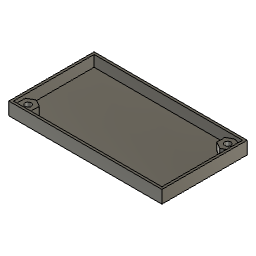
Assemblage v5 (Autodesk Fusion 360 archive; units mm, degrees)
design "Bas"
part number: Configuration1
Autodesk Fusion 360 part; units mm, degrees
sketch "Sketch1" plane through (0, 0, 0) normal (0, 0, 1) x (1, 0, 0)
  line L0 (0, 0) -> (79, 0)
  line L1 (79, 0) -> (79, 44)
  line L2 (79, 44) -> (0, 44)
  line L3 (0, 44) -> (0, 0)
  line L4 (1.2, 1.2) -> (77.8, 1.2)
  line L5 (77.8, 1.2) -> (77.8, 42.8)
  line L6 (77.8, 42.8) -> (1.2, 42.8)
  line L7 (1.2, 42.8) -> (1.2, 1.2)
  line L8 (2, 42) -> (77, 42) construction
  line L9 (77, 42) -> (77, 2) construction
  line L10 (77, 2) -> (2, 2) construction
  line L11 (2, 2) -> (2, 42) construction
  circle A0 centre (74, 39) radius 1.6
  circle A1 centre (5, 5) radius 1.6
  line L12 (74, 42.2332) -> (71.2, 40.6166)
  line L13 (71.2, 40.6166) -> (71.2, 37.3834)
  line L14 (71.2, 37.3834) -> (74, 35.7668)
  line L15 (74, 35.7668) -> (76.8, 37.3834)
  line L16 (76.8, 37.3834) -> (76.8, 40.6166)
  line L17 (76.8, 40.6166) -> (74, 42.2332)
  line L18 (5, 8.2332) -> (2.2, 6.6166)
  line L19 (2.2, 6.6166) -> (2.2, 3.3834)
  line L20 (2.2, 3.3834) -> (5, 1.7668)
  line L21 (5, 1.7668) -> (7.8, 3.3834)
  line L22 (7.8, 3.3834) -> (7.8, 6.6166)
  line L23 (7.8, 6.6166) -> (5, 8.2332)
  line L24 (1.4, 2.9215) -> (5, 0.8431)
  line L25 (5, 0.8431) -> (8.6, 2.9215)
  line L26 (8.6, 2.9215) -> (8.6, 7.0785)
  line L27 (8.6, 7.0785) -> (5, 9.1569)
  line L28 (5, 9.1569) -> (1.4, 7.0785)
  line L29 (1.4, 7.0785) -> (1.4, 2.9215)
  line L30 (70.4, 36.9215) -> (74, 34.8431)
  line L31 (74, 34.8431) -> (77.6, 36.9215)
  line L32 (77.6, 36.9215) -> (77.6, 41.0785)
  line L33 (77.6, 41.0785) -> (74, 43.1569)
  line L34 (74, 43.1569) -> (70.4, 41.0785)
  line L35 (70.4, 41.0785) -> (70.4, 36.9215)
  point P0 (39.5, 42)
  point P1 (39.5, 44)
  point P2 (77, 22)
  point P3 (79, 22)
  point P4 (74, 39)
  point P5 (5, 5)
  dimension "d1" = 79
  dimension "d2" = 44
  dimension "d9" = -1.2
  dimension "d14" = 75
  dimension "d15" = 40
  dimension "d16" = 0.8
  dimension "d21" = 3.2
  dimension "d33" = 2.8
  dimension "d34" = 2.8
  dimension "d35" = 0.8
  dimension "d36" = 0.8
  dimension "d61" = 3.2
  dimension "d63" = 3
  dimension "d64" = 3
  dimension "d65" = 3
  dimension "d66" = 3
  constraint horizontal L0
  constraint vertical L1
  constraint horizontal L2
  constraint vertical L3
  constraint coincident L0.start L3.end
  constraint horizontal L8
  constraint vertical L9
  constraint horizontal L10
  constraint vertical L11
  constraint midpoint L8 P0
  constraint midpoint L2 P1
  constraint vertical P0 P1
  constraint midpoint L9 P2
  constraint midpoint L1 P3
  constraint horizontal P2 P3
  constraint coincident P4 A0.centre
  constraint parallel L5 L16
  constraint coincident P5 A1.centre
  constraint parallel L7 L19
  measures "d1" distance of L1.end L2.end
  measures "d2" distance of L0.end L1.end
  measures "d14" distance of L8.start L8.end
  measures "d15" distance of L8.start L10.end
  measures "d16" distance of L6 L8
  measures "d21" diameter of A0
  measures "d33" distance of P4 L17
  measures "d34" distance of P5 L23
  measures "d61" diameter of A1
  measures "d63" distance of L10 P5
  measures "d64" distance of L11 P5
  measures "d65" distance of L8 P4
  measures "d66" distance of L9 P4
extrude "Extrude13" add sketch "Sketch1" along normal blind 5 contours L12 L13 L14 L15 L16 L17 makes body 1
extrude "Extrude14" add sketch "Sketch1" along normal blind 5 contours L6 L33 L34 | L6 L30 L31 L32 L33 L34 L35 bodies 1
extrude "Extrude15" add sketch "Sketch1" along normal blind 5 separate body contours L4 L24 L25 L26 L27 L28 L29 | L4 L24 L25 | L18 L19 L20 L21 L22 L23 makes body 2
extrude "Extrude16" add sketch "Sketch1" along normal blind 6.6 separate body contours L0 L1 L2 L3 | L4 L24 L25 | L6 L33 L34 makes body 3
extrude "Extrude17" add sketch "Sketch1" along normal blind 0.9 contours L4 L5 L6 L7 L24 L25 L26 L27 L28 L29 L30 L31 L32 L33 L34 L35 bodies 1 2 3
extrude "Extrude18" cut sketch "Sketch1" along normal blind 2.5 contours L12 L13 L14 L15 L16 L17 bodies 1
extrude "Extrude19" cut sketch "Sketch1" along normal blind 2.5 contours L18 L19 L20 L21 L22 L23 bodies 1
sketch "Sketch3" plane through (0, 0, 0) normal (0, 0, 1) x (1, 0, 0)
  line L0 (71.2, 37.4) -> (76.8, 37.4)
  line L1 (76.8, 37.4) -> (74, 35.7468)
  line L2 (74, 35.7468) -> (71.2, 37.4)
  line L3 (71.2, 40.6) -> (76.8, 40.618)
  line L4 (71.2, 40.6) -> (74, 42.2444)
  line L5 (74, 42.2444) -> (76.8, 40.618)
  line L6 (71.2, 37.4) -> (72.4601, 37.4)
  line L7 (2.2, 3.4) -> (7.8, 3.4)
  line L8 (7.8, 3.4) -> (5, 1.7617)
  line L9 (5, 1.7617) -> (2.2, 3.4)
  line L10 (2.2, 6.6) -> (4.9648, 8.2176)
  line L11 (4.9648, 8.2176) -> (7.8, 6.6)
  line L12 (7.8, 6.6) -> (2.2, 6.6)
  constraint horizontal L0
  constraint coincident L0 L6.end
  constraint parallel L0 L7
  constraint parallel L8 L10
  constraint parallel L7 L12
extrude "Extrude20" cut sketch "Sketch3" along normal blind 2.8 contours L7 L8 L9 | L10 L11 L12 bodies 1
extrude "Extrude21" cut sketch "Sketch3" along normal blind 2.8 contours L0 L1 L2 L6 | L3 L4 L5 bodies 1
equation "d1 = TotalDepth"
equation "d2 = TotalWidth"
equation "LayerHeight = 0.3 mm"
equation "Tolerance = 0.1 mm"
equation "ExtrusionWidth = 0.4 mm"
equation "TotalWidth = 44 mm"
equation "TotalDepth = 79 mm"
equation "TotalHeight = 35 mm"
equation "d9 = -3 * ExtrusionWidth"
equation "PCBWidth = 75 mm"
equation "PCBLength = 40 mm"
equation "PCBThickness = 1.6 mm"
equation "PCBSolderingHeight = 4 mm"
equation "d14 = PCBWidth"
equation "d15 = PCBLength"
equation "d21 = M3Adjusted"
equation "M3Adjusted = 3 mm + Tolerance * 2"
equation "PCBSupportHeight = PCBSolderingHeight + Tolerance + BaseThickness"
equation "BottomCaseHeight = PCBSolderingHeight + Tolerance + PCBThickness + BaseThickness"
equation "NutWidth = 5.5 mm + Tolerance"
equation "NutHeight = 2.4 mm + Tolerance"
equation "d33 = NutWidth / 2"
equation "d34 = NutWidth / 2"
equation "d35 = 2 * ExtrusionWidth"
equation "d36 = 2 * ExtrusionWidth"
equation "NutSupportHeight = NutHeight + Tolerance + BaseThickness"
equation "BaseThickness = 3 * LayerHeight"
equation "HoleSpreading = PCBHoleSpread + M3Adjusted / 2"
equation "d61 = M3Adjusted"
equation "PCBHoleSpread = 1.40 mm"
equation "d63 = HoleSpreading"
equation "d64 = HoleSpreading"
equation "d65 = HoleSpreading"
equation "d66 = HoleSpreading"
equation "d67 = PCBSupportHeight"
equation "d69 = PCBSupportHeight"
equation "d71 = PCBSupportHeight"
equation "d73 = BottomCaseHeight"
equation "d75 = BaseThickness"
equation "d77 = NutHeight"
equation "d79 = NutHeight"
equation "d82 = NutHeight + LayerHeight"
equation "d84 = NutHeight + LayerHeight"
